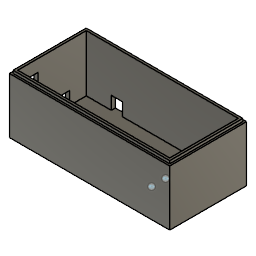
Catlitter (Autodesk Fusion 360 design; units mm, degrees)
part number: 2025-12-03-17-21-55-211
Autodesk Fusion 360 part; units mm, degrees
sketch "Sketch1" plane through (0, 0, 0) normal (0, 0, 1) x (1, 0, 0)
  line L0 (75, -40) -> (-75, -40)
  line L1 (-75, -40) -> (-75, 40)
  line L2 (-75, 40) -> (75, 40)
  line L3 (75, 40) -> (75, -40)
  line L4 (75, -40) -> (-75, 40) construction
  line L5 (-75, -40) -> (75, 40) construction
  dimension "d1" = 150
  dimension "d2" = 80
  constraint horizontal L0
  constraint perpendicular L0 L1
  constraint parallel L0 L2
  constraint parallel L1 L3
  constraint coincident L4 origin
  constraint coincident L5 origin
  measures "d1" distance of L1.end L2.end
  measures "d2" distance of L0.end L1.end
extrude "Extrude1" add sketch "Sketch1" along normal blind 2
sketch "Sketch2" plane through (0, 0, 0) normal (0, 0, -1) x (1, 0, 0)
  line L0 (-75, -40) -> (75, -40)
  line L1 (75, -40) -> (75, 40)
  line L2 (75, 40) -> (-75, 40)
  line L3 (-75, 40) -> (-75, -40)
  line L4 (-76.5, -41.5) -> (76.5, -41.5)
  line L5 (76.5, -41.5) -> (76.5, 41.5)
  line L6 (76.5, 41.5) -> (-76.5, 41.5)
  line L7 (-76.5, 41.5) -> (-76.5, -41.5)
  dimension "d5" = 1.5
extrude "Extrude2" add sketch "Sketch2" against normal blind 60
sketch "Sketch3" plane through (0, 0, 2) normal (0, 0, 1) x (-1, 0, 0)
  line L0 (-75, -40) -> (75, -40)
  line L1 (75, -40) -> (75, 40)
  line L2 (75, 40) -> (-75, 40)
  line L3 (-75, 40) -> (-75, -40)
  circle A0 centre (-45, 5) radius 9.9
  dimension "d8" = 19.8
  measures "d8" diameter of A0
extrude "Extrude3" cut sketch "Sketch3" against normal blind 2 contours A0
sketch "Sketch4" plane through (0, 0, 2) normal (0, 0, 1) x (-1, 0, 0)
  circle A0 centre (-45, 5) radius 9.9
  line L0 (-75, -40) -> (75, -40)
  line L1 (75, -40) -> (75, 40)
  line L2 (75, 40) -> (-75, 40)
  line L3 (-75, 40) -> (-75, -40)
  line L4 (-65, 15) -> (-25, 15)
  line L5 (-25, 15) -> (-25, -5)
  line L6 (-25, -5) -> (-65, -5)
  line L7 (-65, -5) -> (-65, 15)
  line L8 (-65, 15) -> (-25, -5) construction
  line L9 (-25, 15) -> (-65, -5) construction
  line L10 (-26.1043, 0.091) -> (-29.1043, 0.091)
  line L11 (-29.1043, 0.091) -> (-29.1043, 10.091)
  line L12 (-29.1043, 10.091) -> (-26.1043, 10.091)
  line L13 (-26.1043, 10.091) -> (-26.1043, 0.091)
  point P0 (-45, 5)
  dimension "d11" = 40
  dimension "d12" = 20
  dimension "d13" = 3
  dimension "d14" = 10
  constraint horizontal L4
  constraint perpendicular L4 L5
  constraint parallel L4 L6
  constraint parallel L5 L7
  constraint coincident L8 P0
  constraint coincident L9 P0
  constraint coincident P0 A0.centre
  constraint horizontal L10
  constraint vertical L11
  constraint horizontal L12
  constraint vertical L13
  measures "d11" distance of L5.end L6.end
  measures "d12" distance of L4.end L5.end
  measures "d13" distance of L10.start L10.end
  measures "d14" distance of L10.start L12.end
extrude "Extrude4" cut sketch "Sketch4" against normal blind 1 contours L10 L11 L12 L13
sketch "Sketch5" plane through (0, 0, 0) normal (0, 1, 0) x (1, 0, 0)
move_face "OffsetFaces1" offset 3 4 faces at (75, 13.3333, 21.3333) (25, -40, 40.6667) (-25, 40, 40.6667) (-75, -13.3333, 21.3333)
sketch "Sketch6" plane through (0, 37, 0) normal (0, -1, 0) x (1, 0, 0)
  line L0 (-72, 2) -> (72, 2)
  line L1 (72, 2) -> (72, 60)
  line L2 (72, 60) -> (-72, 60)
  line L3 (-72, 60) -> (-72, 2)
  line L4 (-65, 2) -> (-53, 2)
  line L5 (-53, 2) -> (-53, 16)
  line L6 (-53, 16) -> (-65, 16)
  line L7 (-65, 16) -> (-65, 2)
  dimension "d18" = 12
  dimension "d19" = 14
  constraint horizontal L4
  constraint vertical L5
  constraint horizontal L6
  constraint vertical L7
  constraint coincident L0 L4.start
  measures "d18" distance of L4.start L4.end
  measures "d19" distance of L4.start L6.end
extrude "Extrude5" cut sketch "Sketch6" against normal blind 5 contours L0 L4 L5 L6 L7
sketch "Sketch7" plane through (-72, 0, 0) normal (1, 0, 0) x (0, 1, 0)
  line L0 (-37, 2) -> (37, 2)
  line L1 (37, 2) -> (37, 60)
  line L2 (37, 60) -> (-37, 60)
  line L3 (-37, 60) -> (-37, 2)
  line L4 (19, 2) -> (11, 2)
  line L5 (11, 2) -> (11, 8)
  line L6 (11, 8) -> (19, 8)
  line L7 (19, 8) -> (19, 2)
  dimension "d22" = 8
  dimension "d23" = 6
  constraint horizontal L4
  constraint vertical L5
  constraint horizontal L6
  constraint vertical L7
  constraint coincident L0 L4.start
  measures "d22" distance of L4.start L4.end
  measures "d23" distance of L4.start L6.end
extrude "Extrude6" cut sketch "Sketch7" against normal blind 5 contours L0 L4 L5 L6 L7
sketch "Sketch8" plane through (0, 0, 0) normal (0, 1, 0) x (1, 0, 0)
sketch "Sketch9" plane through (0, 0, 60) normal (0, 0, 1) x (-1, 0, 0)
  line L0 (72, 37) -> (72, -37)
  line L1 (72, -37) -> (-72, -37)
  line L2 (-72, -37) -> (-72, 37)
  line L3 (-72, 37) -> (72, 37)
  line L4 (76.5, -41.5) -> (76.5, 41.5)
  line L5 (76.5, 41.5) -> (-76.5, 41.5)
  line L6 (-76.5, 41.5) -> (-76.5, -41.5)
  line L7 (-76.5, -41.5) -> (76.5, -41.5)
  line L8 (74.5, 39.5) -> (-74.5, 39.5)
  line L9 (-74.5, 39.5) -> (-74.5, -39.5)
  line L10 (-74.5, -39.5) -> (74.5, -39.5)
  line L11 (74.5, -39.5) -> (74.5, 39.5)
  dimension "d26" = -2
extrude "Extrude7" add sketch "Sketch9" along normal blind 3 contours L8 L9 L10 L11
sketch "Sketch10" plane through (0, 0, 0) normal (0, 0, 1) x (1, 0, 0)
sketch "Sketch11" plane through (0, 0, 2) normal (0, 0, 1) x (-1, 0, 0)
  circle A0 centre (-28.0143, -2.527) radius 1.5
  circle A1 centre (-28.0453, 12.6041) radius 1.5
  dimension "d29" = 3
  dimension "d30" = 3
  measures "d29" diameter of A0
  measures "d30" diameter of A1
extrude "Extrude8" cut sketch "Sketch11" against normal blind 4 contours A1
extrude "Extrude9" cut sketch "Sketch11" against normal blind 4 contours A0
sketch "Sketch12" plane through (-72, 0, 0) normal (1, 0, 0) x (0, 1, 0)
  line L0 (19, 8) -> (19, 2)
  line L1 (19, 2) -> (37, 2)
  line L2 (37, 2) -> (37, 63)
  line L3 (37, 63) -> (-37, 63)
  line L4 (-37, 63) -> (-37, 2)
  line L5 (-37, 2) -> (11, 2)
  line L6 (11, 2) -> (11, 8)
  line L7 (11, 8) -> (19, 8)
  line L8 (-25, 50) -> (-15, 50)
  line L9 (-15, 50) -> (-15, 40)
  line L10 (-15, 40) -> (-25, 40)
  line L11 (-25, 40) -> (-25, 50)
  constraint horizontal L8
  constraint vertical L9
  constraint horizontal L10
  constraint vertical L11
extrude "Extrude10" cut sketch "Sketch12" against normal blind 5 contours L8 L9 L10 L11
move_face "OffsetFaces2" offset 20 2 faces at (-76.5, 15.1667, 36) (-74.5, 13.1667, 61)
move_face "OffsetFaces3" offset -20 1 faces at (-72, 13.6667, 37)
move_face "OffsetFaces4" offset -8 1 faces at (-93.5, 16.3333, 8)
